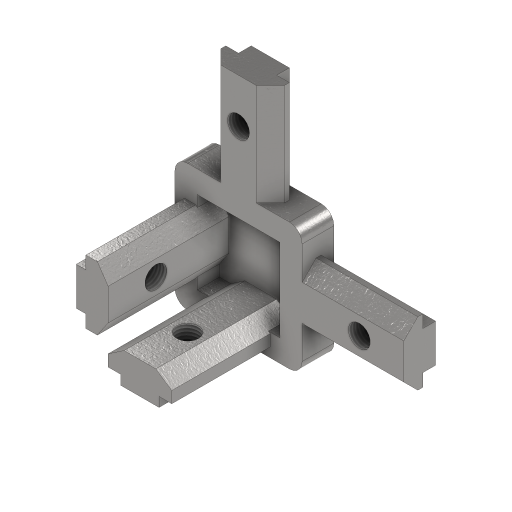
# Autodesk Inventor part: Sambungan Siku
Saved by Autodesk Inventor 2024.4 (Build 284460000, 460)
## iProperties
Created: 2025-10-20
Part Number: Sambungan Siku
Material: Generic
Document SubType Name: Modeling
Designer: Hp
Density: 1 g/cm^3
Appearance: Galvanized
Author: Hp
Autodesk Inventor part; units mm, degrees
ref_plane "YZ Plane" through (0, 0, 0) normal (1, 0, 0) x (0, 1, 0)
ref_plane "XZ Plane" through (0, 0, 0) normal (0, 1, 0) x (-1, 0, 0)
sketch "Sketch1" plane through (0, 0, 0) normal (0, 0, 1) x (1, 0, 0)
  line L0 (10, -10) -> (-10, -10)
  line L1 (-10, -10) -> (-10, 10)
  line L2 (-10, 10) -> (10, 10)
  line L3 (10, 10) -> (10, -10)
  line L4 (10, -10) -> (-10, 10) construction
  line L5 (-10, -10) -> (10, 10) construction
  point P0 (0, 0)
  dimension "d0" = 20
  dimension "d1" = 20
  constraints: 12 end point, 2 midpoint, 2 parallel, 1 horizontal, 1 perpendicular
  measures "d0" distance of L1.end L2.end
  measures "d1" distance of L2.end L0.start
extrude "Extrusion1" add sketch "Sketch1" along normal blind 5
shell "Shell1" thickness 3.5 removed faces 1 at (3.3333, 3.3333, 5)
sketch "Sketch7" plane through (0, 0, 5) normal (0, 0, 1) x (1, 0, 0)
  line L0 (-6.5, -6.5) -> (6.5, -6.5)
  line L1 (6.5, -6.5) -> (6.5, 6.5)
  line L2 (6.5, 6.5) -> (-6.5, 6.5)
  line L3 (-6.5, 6.5) -> (-6.5, -6.5)
  line L4 (-6.5, -6.5) -> (6.5, 6.5) construction
  line L5 (6.5, -6.5) -> (-6.5, 6.5) construction
  line L6 (10, -10) -> (10, 10) projected
  line L7 (-10, -10) -> (10, -10) projected
  point P0 (0, 0)
  dimension "d59" = 3.5
  dimension "d60" = 3.5
  constraints: 12 end point, 2 midpoint, 2 parallel, 1 horizontal, 1 perpendicular
  measures "d59" distance between parallel lines of L6 L1
  measures "d60" distance between parallel lines of L7 L0
extrude "Extrusion5" cut sketch "Sketch7" against normal blind 3.5
sketch "Sketch2" plane through (-6.5, 6.5, 1.5) normal (0, 0, 1) x (1, 0, 0)
  line L0 (9.5, -16.5) -> (3.5, -16.5)
  line L1 (1.5, -15) -> (11.5, -15)
  line L2 (-3.5, -16.5) -> (16.5, -16.5) construction
  line L3 (1.5, -15) -> (1.5, -13.2)
  line L4 (1.5, -13.2) -> (4, -11.5)
  line L5 (4, -11.5) -> (9, -11.5)
  line L6 (9, -11.5) -> (11.5, -13.2)
  line L7 (11.5, -13.2) -> (11.5, -15)
  line L8 (3.5, -15) -> (3.5, -16.5)
  line L9 (9.5, -16.5) -> (9.5, -15)
  point P0 (6.5, -6.5)
  point P1 (6.5, -16.5)
  point P2 (6.5, -16.5)
  point P3 (6.5, -11.5)
  point P4 (6.5, -16.5)
  point P5 (6.5, -15)
  dimension "d6" = 5
  dimension "d7" = 6
  dimension "d9" = 10
  dimension "d10" = 3.5
  dimension "d11" = 1.8
  dimension "d26" = 5
  dimension "d27" = 55.784
  dimension "d63" = 1.5
  constraints: 18 end point, 5 midpoint, 4 point on line, 2 equal length, 2 horizontal, 2 perpendicular, 2 vertical alignment, 1 coincident, 1 collinear, 1 parallel, 1 vertical
  measures "d6" distance of L4.end L5.end
  measures "d7" distance between parallel lines of L8 L9
  measures "d9" distance of L1.start L1.end
  measures "d10" distance between parallel lines of L1 L5
  measures "d11" distance of L6.end L1.end
  measures "d26" distance from line of point (6.5, -6.5) L7
  measures "d27" angle of L7 L6
  measures "d63" distance between parallel lines of L2 L1
extrude "Extrusion2" add sketch "Sketch2" along normal blind 19
sketch "Sketch3" plane through (-2.5, -5, 3.5) normal (0, 1, 0) x (1, 0, 0)
  circle A0 centre (2.5, -9.5) radius 2.5
  line L0 (5, -17) -> (0, -17) construction
  line L1 (12.5, -1.5) -> (-7.5, -1.5) construction
  point P0 (2.5, 3.5)
  point P1 (2.5, -17)
  dimension "d16" = 5
  dimension "d17" = 7.5
  dimension "d18" = 15.5
  constraints: 1 centre point, 1 midpoint, 1 vertical alignment
  measures "d16" diameter of A0
  measures "d17" distance from line of L0 A0.centre
  measures "d18" distance from line of L0.end L1
hole "Hole1" at (0, -5, 13) direction (0, -1, 0) diameter 3.4587 end through all thread size "M4x0.5" class "6H" standard "ANSI Metric M Profile"
ref_plane "Work Plane1" through (-10, -10, 0) normal (-0.7071068, 0.7071068, 0) x (0, 0, -1)
mirror "Mirror1" about plane through (-10, -10, 0) normal (-0.7071068, 0.7071068, 0) of "Extrusion2", "Hole1"
sketch "Sketch4" plane through (-10, 10, 0) normal (0, 1, 0) x (1, 0, 0)
  line L0 (15, -2) -> (15, -2.8)
  line L1 (15, -2.8) -> (12.8, -5)
  line L2 (12.8, -5) -> (7.2, -5)
  line L3 (7.2, -5) -> (5, -2.8)
  line L4 (5, -2.8) -> (5, -2)
  line L5 (14, 0) -> (14, 0)
  line L6 (6, 0) -> (6, 0)
  line L7 (20, 0) -> (0, 0) construction
  line L8 (20, -5) -> (0, -5) construction
  line L9 (15, -2) -> (5, -2)
  line L10 (13, -2) -> (13, 0)
  line L11 (7, -2) -> (7, 0)
  line L12 (13, 0) -> (7, 0)
  point P0 (10, 0)
  point P1 (10, -5)
  point P2 (10, 0)
  point P3 (10, 0)
  point P4 (10, -5)
  point P5 (10, 0)
  point P6 (10, 0)
  point P7 (10, -5)
  point P8 (10, 0)
  point P9 (10, 0)
  point P10 (10, -5)
  point P11 (10, -5)
  point P12 (10, -5)
  point P13 (10, -5)
  point P14 (10, -5)
  point P15 (10, 0)
  point P16 (10, -2)
  point P17 (10, 0)
  dimension "d28" = 5.6
  dimension "d64" = 3
  dimension "d66" = 2
  dimension "d67" = 10
  dimension "d68" = 45
  dimension "d69" = 6
  constraints: 22 end point, 6 vertical alignment, 5 coincident, 2 equal length, 2 midpoint, 2 perpendicular, 2 point on line, 2 vertical, 1 horizontal, 1 parallel, 17 other
  measures "d28" distance of L2.start L3.start
  measures "d64" distance from line of point (10, 0) L11
  measures "d66" distance of the line from the sketch origin of L9
  measures "d67" distance between parallel lines of L0 L4
  measures "d68" angle of L4 L3
  measures "d69" distance between parallel lines of L11 L10
extrude "Extrusion3" add sketch "Sketch4" along normal blind 16
sketch "Sketch5" plane through (0, 0, 5) normal (0, 0, 1) x (1, 0, 0)
  line L0 (-2.8, 26) -> (2.8, 26) construction
  point P0 (0, 0)
  point P1 (0, 19)
  point P2 (0, 26)
  dimension "d41" = 7
  constraints: 1 midpoint, 1 vertical alignment
  measures "d41" distance from line of L0 point (0, 19)
hole "Hole2" at (0, 19, 5) direction (0, 0, -1) diameter 3.4587 end through all thread size "M4x0.5" class "6H" standard "ANSI Metric M Profile"
mirror "Mirror2" about plane through (-10, -10, 0) normal (-0.7071068, 0.7071068, 0) of "Hole2", "Extrusion3"
fillet "Fillet1" radius 2 4 edges at (10, 10, 2.5) (-10, 10, 2.5) (-10, -10, 2.5) (10, -10, 2.5)
equation "\"d1\" = d0"
equation "\"d26\" = 0.5 * d9"
body "Solid1"
